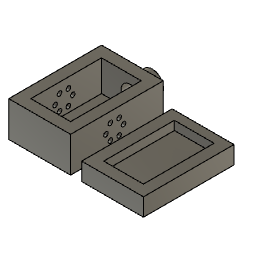
Czujniki v1 (Autodesk Fusion 360 design; units mm, degrees)
Autodesk Fusion 360 part; units mm, degrees
sketch "Sketch1" plane through (0, 0, 0) normal (0, 0, 1) x (1, 0, 0)
  line L0 (-15, 30) -> (3, 30)
  line L1 (3, 30) -> (3, 62)
  line L2 (3, 62) -> (-15, 62)
  line L3 (-15, 62) -> (-15, 30)
  line L4 (8, 67) -> (-20, 67)
  line L5 (-20, 67) -> (-20, 25)
  line L6 (-20, 25) -> (8, 25)
  line L7 (8, 25) -> (8, 67)
  dimension "d1" = 5
  constraint horizontal L0
  constraint vertical L1
  constraint horizontal L2
  constraint vertical L3
extrude "Extrude1" add sketch "Sketch1" along normal blind 16 makes body 1
sketch "Sketch2" plane through (0, 0, 0) normal (0, 0, -1) x (1, 0, 0)
  line L0 (-15, -62) -> (-15, -30)
  line L1 (-15, -30) -> (3, -30)
  line L2 (3, -30) -> (3, -62)
  line L3 (3, -62) -> (-15, -62)
  line L4 (8, -67) -> (8, -25)
  line L5 (8, -25) -> (-20, -25)
  line L6 (-20, -25) -> (-20, -67)
  line L7 (-20, -67) -> (8, -67)
  line L8 (-20, -25) -> (8, -25)
  line L9 (8, -25) -> (8, -67)
  line L10 (8, -67) -> (-20, -67)
  line L11 (-20, -67) -> (-20, -25)
  constraint horizontal L8
  constraint vertical L9
  constraint horizontal L10
  constraint vertical L11
  constraint coincident L4.start L7.end
  constraint coincident L5.end L6.start
extrude "Extrude2" add sketch "Sketch2" against normal blind 2 contours L0 L1 L2 L3 bodies 1
sketch "Sketch3" plane through (0, 67, 0) normal (0, 1, 0) x (-1, 0, 0)
  line L0 (-8, 0) -> (20, 0)
  line L1 (20, 0) -> (20, 16)
  line L2 (20, 16) -> (-8, 16)
  line L3 (-8, 16) -> (-8, 0)
  circle A0 centre (2, 8) radius 4.1231
  circle A1 centre (2, 8) radius 5.1231
  dimension "d8" = 1
extrude "Extrude4" add sketch "Sketch3" along normal blind 5 contours A1 bodies 1
extrude "Extrude3" cut sketch "Sketch3" against normal blind 5 contours A0 bodies 1
sketch "Sketch4" plane through (-20, 0, 0) normal (-1, 0, 0) x (0, -1, 0)
  line L0 (-67, 0) -> (-25, 0)
  line L1 (-25, 0) -> (-25, 16)
  line L2 (-25, 16) -> (-67, 16)
  line L3 (-67, 16) -> (-67, 0)
  circle A0 centre (-41, 8) radius 1.021
  circle A1 centre (-43, 11.4641) radius 1.021
  circle A2 centre (-47, 11.4641) radius 1.021
  circle A3 centre (-49, 8) radius 1.021
  circle A4 centre (-47, 4.5359) radius 1.021
  circle A5 centre (-43, 4.5359) radius 1.021
  point P0 (-45, 8)
  dimension "d12" = 360
extrude "Extrude5" cut sketch "Sketch4" against normal blind 32 contours A0 | A1 | A2 | A3 | A4 | A5 bodies 1
sketch "Sketch5" plane through (0, 0, 0) normal (0, 0, 1) x (1, 0, 0)
  line L0 (13, 25) -> (41, 25)
  line L1 (41, 25) -> (41, 66)
  line L2 (41, 66) -> (13, 66)
  line L3 (13, 66) -> (13, 25)
  constraint horizontal L0
  constraint vertical L1
  constraint horizontal L2
  constraint vertical L3
extrude "Extrude6" add sketch "Sketch5" along normal blind 8 separate body makes body 2
sketch "Sketch6" plane through (0, 0, 8) normal (0, 0, 1) x (-1, 0, 0)
  line L0 (-13, -66) -> (-13, -25)
  line L1 (-13, -25) -> (-41, -25)
  line L2 (-41, -25) -> (-41, -66)
  line L3 (-41, -66) -> (-13, -66)
  line L4 (-18, -62) -> (-36, -62)
  line L5 (-36, -62) -> (-36, -30)
  line L6 (-36, -30) -> (-18, -30)
  line L7 (-18, -30) -> (-18, -62)
  constraint horizontal L4
  constraint vertical L5
  constraint horizontal L6
  constraint vertical L7
extrude "Extrude7" cut sketch "Sketch6" against normal blind 4 contours L4 L5 L6 L7 bodies 2
